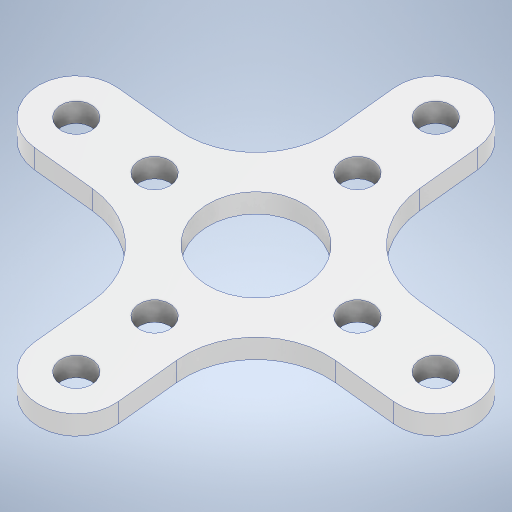
# Autodesk Inventor part: Brushless Motor Mount
Saved by Autodesk Inventor 2024 (Build 280153000, 153)
## iProperties
Created: 2023-10-31
Part Number: Brushless Motor Mount
Material: Generic
Document SubType Name: Modeling
Designer: CJ110
Density: 1 g/cm^3
Appearance: Default
Author: CJ110
Autodesk Inventor part; units mm, degrees
ref_plane "YZ Plane" through (0, 0, 0) normal (1, 0, 0) x (0, 1, 0)
ref_plane "XZ Plane" through (0, 0, 0) normal (0, 1, 0) x (-1, 0, 0)
ref_plane "XY Plane" through (0, 0, 0) normal (0, 0, 1) x (1, 0, 0)
sketch "Sketch1" plane through (0, 0, 0) normal (0, 1, 0) x (-1, 0, 0)
  line L0 (0, 0) -> (30.7, 0)
  line L1 (30.7, 0) -> (30.7, 30.7)
  line L2 (30.7, 30.7) -> (0, 30.7)
  line L3 (0, 30.7) -> (0, 0)
  dimension "d0" = 30.7
  dimension "d1" = 30.7
  constraints: 8 end point, 2 parallel, 1 horizontal, 1 perpendicular
  measures "d0" distance of L2.end L1.end
  measures "d1" distance of L1.end L0.end
extrude "Extrusion1" add sketch "Sketch1" along normal blind 2.032
sketch "Sketch2" plane through (0, 2.032, 0) normal (0, 1, 0) x (1, 0, 0)
  circle A0 centre (-26.89, -26.89) radius 3.81
  circle A1 centre (-3.81, -26.89) radius 3.81
  circle A2 centre (-3.81, -3.81) radius 3.81
  circle A3 centre (-26.89, -3.81) radius 3.81
  circle A4 centre (-15.35, -30.9598) radius 7.2278
  circle A5 centre (-15.35, 0.2598) radius 7.2278
  circle A6 centre (-30.9598, -15.35) radius 7.2278
  circle A7 centre (0.2598, -15.35) radius 7.2278
  line L0 (-29.5841, -24.1959) -> (-25.849, -20.4608)
  line L1 (-25.849, -10.2392) -> (-29.5841, -6.5041)
  line L2 (-24.1959, -1.1159) -> (-20.4608, -4.851)
  line L3 (-10.2392, -4.851) -> (-6.5041, -1.1159)
  line L4 (-1.1159, -6.5041) -> (-4.851, -10.2392)
  line L5 (-4.851, -20.4608) -> (-1.1159, -24.1959)
  line L6 (-6.5041, -29.5841) -> (-10.2392, -25.849)
  line L7 (-20.4608, -25.849) -> (-24.1959, -29.5841)
  line L8 (-30.7, 0) -> (-30.7, -30.7) projected
  line L9 (-30.7, -30.7) -> (0, -30.7) projected
  line L10 (0, -30.7) -> (0, 0) projected
  line L11 (0, 0) -> (-30.7, 0) projected
  line L12 (-23.732, -15.35) -> (-6.968, -15.35) construction
  line L13 (-30.7, -15.35) -> (-23.732, -15.35) construction
  point P0 (-26.89, 0)
  point P1 (-3.81, 0)
  point P2 (-30.7, -3.81)
  point P3 (0, -3.81)
  point P4 (0, -26.89)
  point P5 (-3.81, -30.7)
  point P6 (-26.89, -30.7)
  point P7 (-30.7, -26.89)
  dimension "d4" = 7.62
  dimension "d5" = 16.764
  constraints: 20 end point, 20 tangent, 16 point on circle, 7 centre point, 7 equal length, 3 equal radius, 3 horizontal, 2 parallel, 1 horizontal alignment, 1 midpoint, 1 vertical, 1 vertical alignment, 8 other
  measures "d4" diameter of A0
  measures "d5" distance of L12.start L12.end
extrude "Extrusion2" cut sketch "Sketch2" against normal through all contours A0 L8 A6 L0 | L7 A4 L9 A0 | A0 L9 L8 | A6 L8 | A4 L9 | L6 A1 L9 A4 | L8 A3 L1 A6 | L8 L11 A3 | A1 L10 L9 | L5 A7 L10 A1 | L11 A5 L2 A3 | A7 L10 | L11 A5 | L4 A2 L10 A7 | L11 A2 L3 A5 | L11 L10 A2 picked at (-27.8979, -13.6464) picked at (-16.0496, -27.92) picked at (-4.1409, -17.2716) picked at (-14.1643, -2.5459)
sketch "Sketch3" plane through (0, 2.032, 0) normal (0, 1, 0) x (1, 0, 0)
  circle A0 centre (-26.89, -26.89) radius 1.524
  circle A1 centre (-21.8611, -21.8611) radius 1.524
  circle A2 centre (-15.35, -15.35) radius 4.826
  arc A3 (-29.5841, -24.1959) -> (-24.1959, -29.5841) centre (-26.89, -26.89) ccw projected
  line L0 (-29.5841, -29.5841) -> (0, 0) construction
  line L1 (-25.4985, -30.4368) -> (-30.4368, -25.4985) construction
  line L2 (-18.0893, -23.4775) -> (-23.4775, -18.0893) construction
  arc A4 (-29.5841, -24.1959) -> (-24.1959, -29.5841) centre (-26.89, -26.89) ccw projected
  line L3 (-24.1959, -29.5841) -> (-20.4608, -25.849) projected
  arc A5 (-10.2392, -25.849) -> (-20.4608, -25.849) centre (-15.35, -30.9598) ccw projected
  line L4 (-10.2392, -25.849) -> (-6.5041, -29.5841) projected
  arc A6 (-6.5041, -29.5841) -> (-1.1159, -24.1959) centre (-3.81, -26.89) ccw projected
  line L5 (-1.1159, -24.1959) -> (-4.851, -20.4608) projected
  arc A7 (-4.851, -10.2392) -> (-4.851, -20.4608) centre (0.2598, -15.35) ccw projected
  line L6 (-4.851, -10.2392) -> (-1.1159, -6.5041) projected
  arc A8 (-1.1159, -6.5041) -> (-6.5041, -1.1159) centre (-3.81, -3.81) ccw projected
  line L7 (-6.5041, -1.1159) -> (-10.2392, -4.851) projected
  arc A9 (-20.4608, -4.851) -> (-10.2392, -4.851) centre (-15.35, 0.2598) ccw projected
  line L8 (-20.4608, -4.851) -> (-24.1959, -1.1159) projected
  arc A10 (-24.1959, -1.1159) -> (-29.5841, -6.5041) centre (-26.89, -3.81) ccw projected
  line L9 (-29.5841, -6.5041) -> (-25.849, -10.2392) projected
  arc A11 (-25.849, -20.4608) -> (-25.849, -10.2392) centre (-30.9598, -15.35) ccw projected
  line L10 (-25.849, -20.4608) -> (-29.5841, -24.1959) projected
  line L11 (-29.5841, -1.1159) -> (-1.1159, -29.5841) construction
  circle A12 centre (-3.81, -26.89) radius 1.524
  circle A13 centre (-8.8389, -21.8611) radius 1.524
  circle A14 centre (-3.81, -3.81) radius 1.524
  circle A15 centre (-8.8389, -8.8389) radius 1.524
  circle A16 centre (-26.89, -3.81) radius 1.524
  circle A17 centre (-21.8611, -8.8389) radius 1.524
  dimension "d8" = 3.048
  dimension "d9" = 3.048
  dimension "d10" = 10.16
  dimension "d11" = 9.652
  dimension "d14" = 360
  constraints: 9 centre point, 8 end point, 5 point on circle, 5 point on line, 2 perpendicular, 2 tangent, 1 concentric, 1 midpoint, 17 other
  measures "d8" diameter of A0
  measures "d9" diameter of A1
  measures "d10" distance between parallel lines of L2 L1
  measures "d11" diameter of A2
extrude "Extrusion3" cut sketch "Sketch3" against normal through all contours A0 | A1 | A2 | A12 | A13 | A14 | A15 | A16 | A17
body "Solid1"
